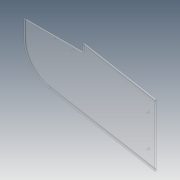
# Autodesk Inventor part: GE-12086-01
Saved by Autodesk Inventor 2012 (Build 160160000, 160)
## iProperties
Created: 2011-10-10
Part Number: GE-12086-01
Document SubType Name: Modeling
Designer: dfoster
Density: 1 g/cm^3
Description: Side
Material: Default
Title: Side
Author: dfoster
Autodesk Inventor part; units mm, degrees
ref_plane "YZ Plane" through (0, 0, 0) normal (1, 0, 0) x (0, 1, 0)
ref_plane "XZ Plane" through (0, 0, 0) normal (0, 1, 0) x (-1, 0, 0)
ref_plane "XY Plane" through (0, 0, 0) normal (0, 0, 1) x (1, 0, 0)
sketch "Sketch1" plane through (0, 0, 0) normal (0, 0, 1) x (1, 0, 0)
  line L0 (0, 0) -> (236.5375, 0)
  line L1 (527.05, 0) -> (527.05, 248.2464)
  line L2 (236.5375, 266.7) -> (0, 266.7)
  line L3 (0, 266.7) -> (0, 195.5132)
  line L4 (527.05, 0) -> (101.0217, 75.1203)
  line L5 (527.05, 248.2464) -> (236.5375, 299.4716)
  line L6 (236.5375, 266.7) -> (236.5375, 299.4716)
  arc A0 (0, 195.5132) -> (101.0217, 75.1203) centre (122.2502, 195.5132) ccw
  circle A1 centre (496.8875, 187.9214) radius 3.3655
  circle A2 centre (496.8875, 60.9214) radius 3.3655
  point P0 (0, 92.9331)
  dimension "d0" = 266.7
  dimension "d2" = 10
  dimension "d3" = 244.475
  dimension "d4" = 236.5375
  dimension "d5" = 527.05
  dimension "d18" = 122.2502
  dimension "d20" = 6.731
  dimension "d21" = 60.325
  dimension "d22" = 127
  dimension "d23" = 30.1625
  dimension "d24" = 30.1625
  constraints: 14 end point, 5 point on line, 4 parallel, 3 centre point, 2 point on circle, 2 tangent, 1 equal radius, 1 horizontal, 1 perpendicular
  measures "d0" distance of L2.end L0.start
  measures "d2" angle of L0 L4
  measures "d3" distance between parallel lines of L5 L4
  measures "d4" distance between parallel lines of L6 L3
  measures "d5" distance between parallel lines of L1 L3
  measures "d18" radius of A0
  measures "d20" diameter of A1
  measures "d21" vertical distance of L1.end A1.centre
  measures "d22" distance of A2.centre A1.centre
  measures "d23" distance from line of L1 A1.centre
  measures "d24" distance from line of L1 A2.centre
extrude "Extrusion1" add sketch "Sketch1" along normal blind 6.35 contours L4 A0 L3 L2 L6 L5 L1 | A1 | A2
sketch "Sketch2" plane through (0, 0, 6.35) normal (0, 0, 1) x (1, 0, 0)
  line L0 (236.5375, 266.7) -> (236.5375, 299.4716) projected
  line L1 (0, 266.7) -> (236.5375, 266.7) projected
  line L2 (0, 195.5132) -> (0, 266.7) projected
  line L3 (527.05, 0) -> (101.0217, 75.1203) projected
  line L4 (527.05, 248.2464) -> (527.05, 0) projected
  line L5 (236.5375, 299.4716) -> (527.05, 248.2464) projected
  line L6 (236.5375, 294.6227) -> (527.05, 243.3976)
  line L7 (527.05, 4.8489) -> (101.8509, 79.8229)
  line L8 (4.7752, 195.5132) -> (4.7752, 266.7)
  line L9 (236.5375, 291.3988) -> (527.05, 240.1736)
  line L10 (527.05, 8.0728) -> (102.4022, 82.9497)
  line L11 (7.9502, 195.5132) -> (7.9502, 266.7)
  line L12 (4.7752, 266.7) -> (7.9502, 266.7)
  line L13 (527.05, 8.0728) -> (527.05, 4.8489)
  line L14 (236.5375, 294.6227) -> (236.5375, 291.3988)
  line L15 (527.05, 243.3976) -> (527.05, 240.1736)
  arc A0 (7.9502, 195.5132) -> (102.4022, 82.9497) centre (122.2502, 195.5132) ccw
  arc A1 (4.7752, 195.5132) -> (101.8509, 79.8229) centre (122.2502, 195.5132) ccw
  point P0 (0, 88.4544)
  point P1 (0, 0)
  point P2 (4.7752, 96.94)
  point P3 (7.9502, 99.6041)
  point P4 (101.0217, 75.1203)
  dimension "d8" = 3.175
  dimension "d9" = 4.7752
  dimension "d10" = 4.7752
  dimension "d11" = 3.175
  dimension "d12" = 4.7752
  dimension "d13" = 3.175
  dimension "d16" = 114.3
  dimension "d17" = 117.475
  constraints: 20 end point, 12 point on line, 4 point on circle, 4 tangent, 2 centre point, 2 collinear, 1 perpendicular, 1 other
  measures "d8" distance between parallel lines of L11 L8
  measures "d9" distance between parallel lines of L8 L2
  measures "d11" distance between parallel lines of L10 L7
  measures "d12" distance between parallel lines of L6 L5
  measures "d13" distance between parallel lines of L9 L6
  measures "d16" radius of A0
  measures "d17" radius of A1
extrude "Extrusion2" cut sketch "Sketch2" against normal blind 3.175 contours L0 L6 L4 L9 | L11 A0 L10 L4 L7 A1 L8 L1
extrude "Extrusion3" cut sketch "Sketch1" along normal blind 25.4 contours A1 | A2
hole "Hole1" at (41.275, 254, 6.35) direction (0, 0, -1) diameter 6.35 depth 25.4 tip angle 118
pattern_linear "Rectangular Pattern1" count 3 spacing 76.2 along (1, 0, 0) of "Hole1"
equation "\"d24\" = d23"
body "Solid1"
